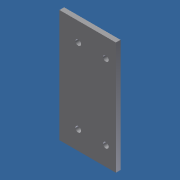
# Autodesk Inventor part: front frame plate
Saved by Autodesk Inventor 2012 (Build 160160000, 160)
## iProperties
Created: 2012-03-16
Part Number: front frame plate
Material: Default
Document SubType Name: Modeling
Designer: Ed
Density: 1 g/cm^3
Author: Ed
Autodesk Inventor part; units mm, degrees
ref_plane "YZ Plane" through (0, 0, 0) normal (1, 0, 0) x (0, 1, 0)
ref_plane "XZ Plane" through (0, 0, 0) normal (0, 1, 0) x (-1, 0, 0)
ref_plane "XY Plane" through (0, 0, 0) normal (0, 0, 1) x (1, 0, 0)
sketch "Sketch1" plane through (0, 0, 0) normal (0, 0, 1) x (1, 0, 0)
  line L0 (0, 0) -> (76.2, 0)
  line L1 (76.2, 0) -> (76.2, 152.4)
  line L2 (76.2, 152.4) -> (0, 152.4)
  line L3 (0, 152.4) -> (0, 0)
  dimension "d0" = 152.4
  dimension "d1" = 76.2
  constraints: 8 end point, 2 parallel, 1 horizontal, 1 perpendicular
  measures "d0" distance of L2.end L0.start
  measures "d1" distance of L0.start L0.end
extrude "Extrusion1" add sketch "Sketch1" along normal blind 6.35
sketch "Sketch2" plane through (0, 0, 6.35) normal (0, 0, 1) x (1, 0, 0)
  line L0 (0, 0) -> (0, 152.4) projected
  line L1 (76.2, 0) -> (0, 0) projected
  line L2 (76.2, 152.4) -> (76.2, 0) projected
  point P0 (25.4, 127)
  point P1 (62.7126, 127)
  point P2 (62.7126, 25.4)
  point P3 (25.4, 25.4)
  dimension "d4" = 101.6
  dimension "d5" = 25.4
  dimension "d7" = 25.4
  dimension "d8" = 13.4874
  constraints: 2 horizontal alignment, 2 vertical alignment
  measures "d4" distance of point (25.4, 127) point (25.4, 25.4)
  measures "d5" distance from line of L0 point (25.4, 25.4)
  measures "d7" distance from line of L1 point (25.4, 25.4)
  measures "d8" distance from line of L2 point (62.713, 25.4)
hole "Hole1" at (25.4, 127, 6.35) at (62.7126, 127, 6.35) at (62.7126, 25.4, 6.35) at (25.4, 25.4, 6.35) direction (0, 0, -1) diameter 7.62 end through all
body "Solid1"
